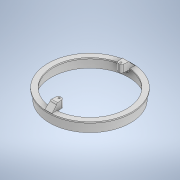
# Autodesk Inventor part: gripper_mount_ring
Saved by Autodesk Inventor 2022 (Build 260153000, 153)
## iProperties
Created: 2022-03-15
Part Number: gripper_mount_ring
Material: Generic
Document SubType Name: Modeling
Designer: kylem
Density: 1 g/cm^3
Appearance: Default
Author: kylem
Autodesk Inventor part; units mm, degrees
ref_plane "YZ Plane" through (0, 0, 0) normal (1, 0, 0) x (0, 1, 0)
ref_plane "XZ Plane" through (0, 0, 0) normal (0, 1, 0) x (-1, 0, 0)
ref_plane "XY Plane" through (0, 0, 0) normal (0, 0, 1) x (1, 0, 0)
sketch "Sketch1" plane through (0, 0, 0) normal (0, 1, 0) x (-1, 0, 0)
  circle A0 centre (0, 0) radius 65.5
  circle A1 centre (0, 0) radius 62.5
  dimension "d0" = 131
  dimension "d1" = 125
  constraints: 2 centre point, 2 coincident
  measures "d0" diameter of A0
  measures "d1" diameter of A1
extrude "Extrusion1" add sketch "Sketch1" along normal blind 15
sketch "Sketch2" plane through (0, 15, 0) normal (0, 1, 0) x (1, 0, 0)
  line L0 (0, 0) -> (1.9, 0)
  line L1 (1.9, 0) -> (-1.9, 0)
  line L2 (-1.9, 0) -> (-1.9, 75.6091)
  line L3 (-1.9, 75.6091) -> (1.9, 75.6091)
  line L4 (1.9, 75.6091) -> (1.9, 0)
  line L5 (1.9, 75.6091) -> (-1.9, 75.6091)
  line L6 (-1.9, 75.6091) -> (-1.9, -80.0242)
  line L7 (-1.9, -80.0242) -> (1.9, -80.0242)
  line L8 (1.9, -80.0242) -> (1.9, 75.6091)
  circle A0 centre (0, 0) radius 62.5 projected
  circle A1 centre (0, 0) radius 62.5
  circle A2 centre (0, 0) radius 59.5
  point P0 (-1.9, 59.4697)
  point P1 (1.9, 59.4697)
  point P2 (1.9, 62.4711)
  point P3 (-1.9, 62.4711)
  point P4 (1.9, -59.4697)
  point P5 (-1.9, -59.4697)
  point P6 (-1.9, -62.4711)
  point P7 (1.9, -62.4711)
  dimension "d4" = 1.9
  dimension "d5" = 3.8
  dimension "d6" = 3.8
  dimension "d7" = 119
  constraints: 18 end point, 4 parallel, 3 horizontal, 2 centre point, 2 coincident, 2 perpendicular
  measures "d4" distance of L0.start L0.end
  measures "d5" distance of L2.end L3.end
  measures "d6" distance of L7.end L6.end
  measures "d7" diameter of A2
extrude "Extrusion2" add sketch "Sketch2" against normal blind 7.5 contours A2 L2 A0 L4 | L8 A0 L6 A2
chamfer "Chamfer3" distance 1.8 angle 45 4 edges at (1.9, 7.5, -60.9704) (-1.9, 7.5, -60.9704) (1.9, 7.5, 60.9704) (-1.9, 7.5, 60.9704)
sketch "Sketch4" plane through (0, 15, 0) normal (0, 1, 0) x (1, 0, 0)
  line L0 (1.9, 59.4697) -> (1.9, 62.4711) projected
  circle A0 centre (0, 0) radius 59.5
  circle A1 centre (0, 0) radius 68
  arc A2 (-0.1, 59.4999) -> (-1.9, 59.4697) centre (0, 0) ccw projected
  line L1 (1.9, 62.4711) -> (-1.9, 62.4711)
  line L2 (-1.9, 62.4711) -> (-1.9, 59.4697)
  line L3 (-1.9, 59.4697) -> (1.9, 59.4697)
  line L4 (1.9, 59.4697) -> (1.9, 62.4711)
  line L5 (-1.9, -62.4711) -> (-1.9, -59.4697) projected
  arc A3 (0.1, -59.4999) -> (1.9, -59.4697) centre (0, 0) ccw projected
  line L6 (-1.9, -62.4711) -> (1.9, -62.4711)
  line L7 (1.9, -62.4711) -> (1.9, -59.4697)
  line L8 (1.9, -59.4697) -> (-1.9, -59.4697)
  line L9 (-1.9, -59.4697) -> (-1.9, -62.4711)
  dimension "d22" = 136
  constraints: 16 end point, 4 parallel, 2 centre point, 2 coincident, 2 horizontal, 2 perpendicular, 1 point on circle
  measures "d22" diameter of A1
extrude "Extrusion3" add sketch "Sketch4" along normal blind 2
sketch "Sketch5" plane through (0, 17, 0) normal (0, 1, 0) x (1, 0, 0)
  arc A0 (1.9, -59.4697) -> (1.9, 59.4697) centre (0, 0) ccw projected
  circle A1 centre (0, 0) radius 59.5
  circle A2 centre (0, 0) radius 62.5
  line L0 (-0.1, 62.4999) -> (-0.1, 59.4999) projected
  line L1 (-0.1, 62.4999) -> (-0.1, 52.9291)
  circle A3 centre (-0.1, 52.9291) radius 1.375
  line L2 (0, 0) -> (7.9858, 0)
  circle A4 centre (-0.1, -52.9291) radius 1.375
  line L3 (0, 0) -> (5.1858, 59.2736)
  line L4 (0, 0) -> (59.5, 0) construction
  line L5 (0, 0) -> (0, 22.2249)
  line L6 (0, 0) -> (-5.1858, 59.2736)
  line L7 (0, 0) -> (5.1858, -59.2736)
  line L8 (0, 0) -> (-5.1858, -59.2736)
  circle A5 centre (0, 0) radius 59.5
  circle A6 centre (0, 0) radius 59.5
  circle A7 centre (0, 0) radius 45
  point P0 (-3.922, 44.8288)
  point P1 (3.922, 44.8288)
  point P2 (3.922, -44.8288)
  point P3 (-3.922, -44.8288)
  point P4 (1.9, -59.4697)
  dimension "d25" = 125
  dimension "d26" = 2.75
  dimension "d28" = 59.5
  dimension "d29" = 85
  dimension "d30" = 90
  constraints: 16 end point, 6 coincident, 4 centre point, 4 symmetric about line, 2 horizontal, 2 vertical, 1 equal length, 1 point on circle, 9 other
  measures "d26" diameter of A3
  measures "d28" distance of L2.start L3.end
  measures "d29" angle of L4 L3
  measures "d30" diameter of A7
extrude "Extrusion4" add sketch "Sketch5" along normal blind 10 contours A1 L8 A7 L7 A0 | A1 A0 L3 A7 L6
extrude "Extrusion5" add sketch "Sketch4" along normal blind 2 contours A0 L2 L1 L0 | L7 L6 L5 A0
extrude "Extrusion6" add sketch "Sketch5" against normal blind 2 contours A1 L8 A7 L7 A0 | A1 A0 L3 A7 L6
chamfer "Chamfer4" distance 8 angle 45 2 edges at (0, 17, -59.5) (0, 17, 59.5)
fillet "Fillet1" radius 2 2 edges at (0, 27, -59.5) (0, 27, 59.5)
sketch "Sketch6" plane through (0, 15, 0) normal (0, -1, 0) x (1, 0, 0)
  circle A0 centre (-0.1, -52.9291) radius 1.375 projected
  circle A1 centre (-0.1, -52.9291) radius 1.375
  circle A2 centre (-0.1, 52.9291) radius 1.375 projected
  circle A3 centre (-0.1, 52.9291) radius 1.375
  point P0 (0, 0)
  constraints: 2 centre point, 2 coincident
extrude "Extrusion7" add sketch "Sketch6" against normal blind 12
sketch "Sketch7" plane through (0, 15, 0) normal (0, -1, 0) x (1, 0, 0)
  arc A0 (3.922, 44.8288) -> (-3.922, 44.8288) centre (0, 0) ccw projected
  line L0 (0, 0) -> (0, -50)
  circle A1 centre (0, -50) radius 1.375
  line L1 (0, 0) -> (-11.0187, 0)
  circle A2 centre (0, 50) radius 1.375
  point P0 (0.9264, -44.9905)
  point P1 (-0.9264, -44.9905)
  dimension "d46" = 50
  dimension "d47" = 2.75
  constraints: 4 end point, 2 centre point, 1 coincident, 1 horizontal, 1 symmetric about line, 1 vertical, 1 other
  measures "d46" distance of L0.start L0.end
  measures "d47" diameter of A1
extrude "Extrusion8" cut sketch "Sketch7" against normal blind 12
sketch "Sketch8" plane through (0, 15, 0) normal (0, -1, 0) x (1, 0, 0)
  circle A0 centre (0, 0) radius 47
  dimension "d50" = 94
  constraints: 1 centre point, 1 coincident
  measures "d50" diameter of A0
extrude "Extrusion9" cut sketch "Sketch8" against normal blind 12
fillet "Fillet2" radius 3 4 edges at (4.0963, 21, -46.8212) (-4.0963, 21, -46.8212) (4.0963, 21, 46.8212) (-4.0963, 21, 46.8212)
body "Solid1"
